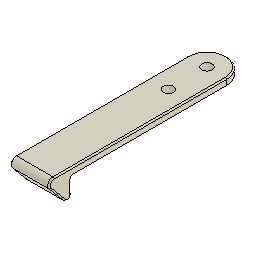
domingo-fermentor-v0-3-cabinet-200 (Autodesk Fusion 360 archive; units mm, degrees)
design "door_lock"
Autodesk Fusion 360 part; units mm, degrees
note: some values were not read from the file. Chosen so that the rebuilt part matches the saved one: which face or edge a step refers to. Set by a fixed rule: which sketch regions a step uses.
sketch "Sketch1" plane through (0, 0, 0) normal (0, 0, 1) x (1, 0, 0)
  line L0 (-7.5, 30) -> (7.5, 30) construction
  line L1 (7.5, 30) -> (7.5, -30)
  line L2 (7.5, -30) -> (-7.5, -30)
  line L3 (-7.5, -30) -> (-7.5, 30)
  line L4 (0, 30) -> (0, -30) construction
  line L5 (-7.5, 0) -> (7.5, 0) construction
  arc A0 (7.5, 30) -> (-7.5, 30) centre (0, 30) ccw
  circle A1 centre (0, 30) radius 2
  circle A2 centre (0, 15) radius 2
  line L6 (-7.5, -30) -> (7.5, -30)
  line L7 (7.5, -30) -> (7.5, -43)
  line L8 (7.5, -43) -> (-7.5, -43)
  line L9 (-7.5, -43) -> (-7.5, -30)
  point P0 (20, 20)
  dimension "d5" = 15
  dimension "d6" = 60
  dimension "d7" = 4
  dimension "d8" = 4
  dimension "d9" = 15
  dimension "d10" = 13
  constraint horizontal L0
  constraint vertical L1
  constraint horizontal L2
  constraint vertical L3
  constraint midpoint L0 L4.start
  constraint midpoint L2 L4.end
  constraint midpoint L3 L5.start
  constraint midpoint L1 L5.end
  constraint midpoint L4 origin
  constraint coincident L4.start A0.centre
  constraint concentric A0 A1
  constraint coincident L4 A2.centre
  constraint horizontal L6
  constraint vertical L7
  constraint horizontal L8
  constraint vertical L9
  constraint equal L0 L8
  measures "d5" distance of L0.start L0.end
  measures "d6" distance of L0.start L2.end
  measures "d7" diameter of A1
  measures "d8" diameter of A2
  measures "d9" distance of L4.start A2.centre
  measures "d10" distance of L2.end L8.end
extrude "Extrude1" add sketch "Sketch1" along normal blind 3 makes body 1
sketch "Sketch2" plane through (7.5, 0, 0) normal (1, 0, 0) x (0, 1, 0)
  line L0 (-43, 0) -> (30, 0)
  line L1 (30, 0) -> (30, 3)
  line L2 (30, 3) -> (-43, 3)
  line L3 (-43, 3) -> (-43, 0)
  line L4 (-30, 0) -> (-30, -10)
  line L5 (-30, -10) -> (2.0156, -10) construction
  line L6 (-43, 3) -> (-30, 3)
  line L7 (-30, 0) -> (-30, 3)
  line L8 (-30, -10) -> (-110.3485, 85.7556)
  line L9 (-30, -10) -> (95, -10) construction
  dimension "d13" = 10
  dimension "d27" = 130
  dimension "d28" = 125
  constraint coincident L0 L4.start
  constraint perpendicular L0 L4
  constraint horizontal L5
  constraint coincident L2.end L3.start
  constraint coincident L2 L6.end
  constraint perpendicular L3 L6
  constraint horizontal L9
  measures "d13" distance of L4.start L4.end
  measures "d27" angle of L8 L9
  measures "d28" distance of L4.end L8.end
extrude "Extrude2" add sketch "Sketch2" against normal blind 15 separate body contours L0 L4 L8 makes body 2
extrude "Extrude3" cut sketch "Sketch2" against normal blind 15 contours L0 L2 L3 L6 L8 bodies 1
combine "Combine1" operation add target body 2 tool bodies 1
fillet "Fillet1" radius 2 1 edges at (0, -40.9083, 3) on bodies 2
fillet "Fillet2" radius 1.5 1 edges at (0, -30, -10) on bodies 2
fillet "Fillet3" radius 0.5 1 edges at (0, -30, 0) on bodies 2
fillet "Fillet4" radius 0.5 16 edges at (-7.5, -30, -3.1894) (-7.5, -29.8536, -0.1464) (-7.5, -30.987, -7.2883) (-7.5, 0.25, 0) (-7.5, -35.4002, -3.5643) (-7.5, -38.4319, 1.8452) (-7.5, -3.3096, 3) (7.5, -30, -3.1894) (7.5, -29.8536, -0.1464) (7.5, -30.987, -7.2883) (0, 37.5, 0) (7.5, 0.25, 0) (7.5, -35.4002, -3.5643) (0, 37.5, 3) (7.5, -38.4319, 1.8452) (7.5, -3.3096, 3) on bodies 2
equation "lock_width = 15 mm"
equation "lock_lenght = 60 mm"
equation "lock_tickness = 3 mm"
equation "lock_fold = 10 mm"
equation "d5 = lock_width"
equation "d6 = lock_lenght"
equation "d11 = lock_tickness"
equation "d13 = lock_fold"
equation "d15 = -lock_width"
equation "d17 = -lock_width"
